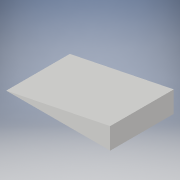
# Autodesk Inventor part: Ramp
Saved by Autodesk Inventor 2017 (Build 210142000, 142)
## iProperties
Created: 2017-04-14
Part Number: Ramp
Material: Generic
Document SubType Name: Modeling
Designer: Alex Tacescu
Density: 1 g/cm^3
Appearance: Default
Author: Alex Tacescu
Autodesk Inventor part; units mm, degrees
ref_plane "YZ Plane" through (0, 0, 0) normal (1, 0, 0) x (0, 1, 0)
ref_plane "XZ Plane" through (0, 0, 0) normal (0, 1, 0) x (-1, 0, 0)
ref_plane "XY Plane" through (0, 0, 0) normal (0, 0, 1) x (1, 0, 0)
sketch "Sketch1" plane through (0, 0, 0) normal (0, 0, 1) x (1, 0, 0)
  line L0 (0, 0) -> (746.6045, 152.4)
  line L1 (0, 182.88) -> (0, -30.48) projected
  line L2 (-149.3209, 0) -> (895.9254, 0) projected
  line L3 (746.6045, 152.4) -> (746.6045, 0)
  line L4 (0, 0) -> (746.6045, 0)
  dimension "d0" = 152.4
  dimension "d1" = 762
  constraints: 6 end point, 1 perpendicular, 1 point on line, 1 vertical
  measures "d0" distance of L0.end L3.end
  measures "d1" distance of L0.start L0.end
extrude "Extrusion1" add sketch "Sketch1" along normal mid plane 457.2
body "Solid1"
